Autodesk Fusion 360 part; units mm, degrees
(part 2 of 3)
  spline S18 degree 5 poles (-4.419, 9.1361) (-4.4209, 9.1399) (-4.4247, 9.1474) (-4.4306, 9.1586) (-4.439, 9.1732) (-4.4502, 9.1911) (-4.4619, 9.2087) (-4.4739, 9.2262) (-4.4861, 9.2436) (-4.4984, 9.2609) (-4.5108, 9.2782) (-4.5234, 9.2954) (-4.5362, 9.3124) (-4.5493, 9.3294) (-4.5626, 9.3462) (-4.5761, 9.3629) (-4.5898, 9.3794) (-4.6036, 9.3959) (-4.6176, 9.4123) (-4.6318, 9.4286) (-4.6461, 9.4449) (-4.6605, 9.461) (-4.6751, 9.4771) (-4.6898, 9.4931) (-4.7046, 9.509) (-4.7196, 9.5248) (-4.7348, 9.5406) (-4.75, 9.5562) (-4.7654, 9.5718) (-4.7809, 9.5873) (-4.7966, 9.6027) (-4.8123, 9.6181) (-4.8282, 9.6334) (-4.8442, 9.6486) (-4.8603, 9.6637) (-4.8765, 9.6788) (-4.8929, 9.6938) (-4.9093, 9.7087) (-4.9259, 9.7236) (-4.9425, 9.7384) (-4.9593, 9.7531) (-4.9762, 9.7677) (-4.9931, 9.7823) (-5.0102, 9.7968) (-5.0274, 9.8112) (-5.0447, 9.8256) (-5.0621, 9.8399) (-5.0796, 9.8541) (-5.0971, 9.8683) (-5.1148, 9.8824) (-5.1326, 9.8964) (-5.1505, 9.9103) (-5.1684, 9.9242) (-5.1865, 9.9381) (-5.2046, 9.9518) (-5.2229, 9.9655) (-5.2412, 9.9791) (-5.2596, 9.9927) (-5.2781, 10.0062) (-5.2967, 10.0196) (-5.3154, 10.033) (-5.3342, 10.0463) (-5.353, 10.0595) (-5.3719, 10.0727) (-5.391, 10.0858) (-5.4101, 10.0988) (-5.4293, 10.1118) (-5.4486, 10.1247) (-5.4679, 10.1375) (-5.4874, 10.1503) (-5.5069, 10.163) (-5.5226, 10.1731) (-5.5344, 10.1807) (-5.5422, 10.1857) (-5.5462, 10.1882) knots 0 0 0 0 0 0 0.01428571 0.02857143 0.04285714 0.05714286 0.07142857 0.08571429 0.1 0.11428571 0.12857143 0.14285714 0.15714286 0.17142857 0.18571429 0.2 0.21428571 0.22857143 0.24285714 0.25714286 0.27142857 0.28571429 0.3 0.31428571 0.32857143 0.34285714 0.35714286 0.37142857 0.38571429 0.4 0.41428571 0.42857143 0.44285714 0.45714286 0.47142857 0.48571429 0.5 0.51428571 0.52857143 0.54285714 0.55714286 0.57142857 0.58571429 0.6 0.61428571 0.62857143 0.64285714 0.65714286 0.67142857 0.68571429 0.7 0.71428571 0.72857143 0.74285714 0.75714286 0.77142857 0.78571429 0.8 0.81428571 0.82857143 0.84285714 0.85714286 0.87142857 0.88571429 0.9 0.91428571 0.92857143 0.94285714 0.95714286 0.97142857 0.98571429 1 1 1 1 1 1
  arc A38 (-5.5462, 10.1882) -> (-6.0502, 9.8972) centre (0, 0) ccw
  spline S19 degree 5 poles (-6.0502, 9.8972) (-6.05, 9.8926) (-6.0496, 9.8832) (-6.0489, 9.8692) (-6.048, 9.8506) (-6.0467, 9.8273) (-6.0454, 9.8041) (-6.044, 9.7809) (-6.0424, 9.7578) (-6.0408, 9.7347) (-6.039, 9.7116) (-6.0372, 9.6886) (-6.0353, 9.6656) (-6.0333, 9.6426) (-6.0311, 9.6197) (-6.0289, 9.5969) (-6.0266, 9.5741) (-6.0241, 9.5513) (-6.0216, 9.5286) (-6.019, 9.5059) (-6.0162, 9.4832) (-6.0134, 9.4606) (-6.0104, 9.4381) (-6.0074, 9.4156) (-6.0042, 9.3931) (-6.001, 9.3707) (-5.9976, 9.3484) (-5.9941, 9.3261) (-5.9905, 9.3038) (-5.9868, 9.2816) (-5.9831, 9.2595) (-5.9791, 9.2374) (-5.9751, 9.2153) (-5.971, 9.1933) (-5.9668, 9.1714) (-5.9624, 9.1495) (-5.9579, 9.1277) (-5.9533, 9.1059) (-5.9486, 9.0842) (-5.9438, 9.0626) (-5.9389, 9.041) (-5.9338, 9.0195) (-5.9287, 8.998) (-5.9234, 8.9767) (-5.9179, 8.9553) (-5.9124, 8.9341) (-5.9067, 8.9129) (-5.9009, 8.8918) (-5.895, 8.8707) (-5.8889, 8.8497) (-5.8827, 8.8288) (-5.8764, 8.808) (-5.8699, 8.7873) (-5.8632, 8.7666) (-5.8565, 8.7461) (-5.8495, 8.7256) (-5.8425, 8.7052) (-5.8353, 8.6848) (-5.8279, 8.6646) (-5.8204, 8.6444) (-5.8128, 8.6244) (-5.8048, 8.6045) (-5.7967, 8.5847) (-5.7883, 8.5651) (-5.7797, 8.5456) (-5.771, 8.5262) (-5.7622, 8.5068) (-5.7532, 8.4876) (-5.7441, 8.4685) (-5.7346, 8.4495) (-5.7247, 8.4309) (-5.7163, 8.4163) (-5.7095, 8.4056) (-5.7049, 8.3985) (-5.7025, 8.395) knots -1 -1 -1 -1 -1 -1 -0.98571429 -0.97142857 -0.95714286 -0.94285714 -0.92857143 -0.91428571 -0.9 -0.88571429 -0.87142857 -0.85714286 -0.84285714 -0.82857143 -0.81428571 -0.8 -0.78571429 -0.77142857 -0.75714286 -0.74285714 -0.72857143 -0.71428571 -0.7 -0.68571429 -0.67142857 -0.65714286 -0.64285714 -0.62857143 -0.61428571 -0.6 -0.58571429 -0.57142857 -0.55714286 -0.54285714 -0.52857143 -0.51428571 -0.5 -0.48571429 -0.47142857 -0.45714286 -0.44285714 -0.42857143 -0.41428571 -0.4 -0.38571429 -0.37142857 -0.35714286 -0.34285714 -0.32857143 -0.31428571 -0.3 -0.28571429 -0.27142857 -0.25714286 -0.24285714 -0.22857143 -0.21428571 -0.2 -0.18571429 -0.17142857 -0.15714286 -0.14285714 -0.12857143 -0.11428571 -0.1 -0.08571429 -0.07142857 -0.05714286 -0.04285714 -0.02857143 -0.01428571 0 0 0 0 0 0
  line L19 (-5.7025, 8.395) -> (-5.5568, 8.1795)
  arc A39 (-5.5826, 8.0414) -> (-5.5568, 8.1795) centre (-5.6396, 8.1235) ccw
  arc A40 (-5.5826, 8.0414) -> (-6.1024, 7.6543) centre (0, 0) ccw
  arc A41 (-6.2422, 7.6692) -> (-6.1024, 7.6543) centre (-6.1648, 7.7325) ccw
  line L20 (-6.2422, 7.6692) -> (-6.4069, 7.8707)
  spline S20 degree 5 poles (-6.4069, 7.8707) (-6.4095, 7.874) (-6.4149, 7.8804) (-6.4233, 7.8899) (-6.4348, 7.9022) (-6.4498, 7.9171) (-6.4653, 7.9315) (-6.481, 7.9458) (-6.4969, 7.9599) (-6.5128, 7.9739) (-6.5289, 7.9878) (-6.5451, 8.0016) (-6.5615, 8.0153) (-6.5781, 8.0288) (-6.5949, 8.0421) (-6.6119, 8.0552) (-6.6291, 8.0681) (-6.6464, 8.081) (-6.6638, 8.0937) (-6.6813, 8.1063) (-6.699, 8.1188) (-6.7167, 8.1312) (-6.7346, 8.1435) (-6.7526, 8.1557) (-6.7707, 8.1677) (-6.789, 8.1797) (-6.8073, 8.1915) (-6.8258, 8.2032) (-6.8444, 8.2148) (-6.8631, 8.2263) (-6.8818, 8.2377) (-6.9007, 8.249) (-6.9197, 8.2603) (-6.9387, 8.2714) (-6.9579, 8.2824) (-6.9772, 8.2933) (-6.9965, 8.3041) (-7.016, 8.3149) (-7.0355, 8.3255) (-7.0551, 8.336) (-7.0748, 8.3465) (-7.0946, 8.3568) (-7.1145, 8.3671) (-7.1345, 8.3773) (-7.1545, 8.3873) (-7.1746, 8.3973) (-7.1949, 8.4072) (-7.2152, 8.4171) (-7.2355, 8.4268) (-7.256, 8.4364) (-7.2765, 8.446) (-7.2971, 8.4554) (-7.3178, 8.4648) (-7.3385, 8.4741) (-7.3594, 8.4833) (-7.3803, 8.4924) (-7.4012, 8.5014) (-7.4223, 8.5104) (-7.4434, 8.5193) (-7.4646, 8.528) (-7.4859, 8.5367) (-7.5072, 8.5453) (-7.5286, 8.5539) (-7.5501, 8.5623) (-7.5716, 8.5707) (-7.5932, 8.5789) (-7.6149, 8.5871) (-7.6366, 8.5952) (-7.6584, 8.6033) (-7.6803, 8.6112) (-7.7022, 8.6191) (-7.7198, 8.6253) (-7.733, 8.63) (-7.7418, 8.633) (-7.7462, 8.6346) knots 0 0 0 0 0 0 0.01428571 0.02857143 0.04285714 0.05714286 0.07142857 0.08571429 0.1 0.11428571 0.12857143 0.14285714 0.15714286 0.17142857 0.18571429 0.2 0.21428571 0.22857143 0.24285714 0.25714286 0.27142857 0.28571429 0.3 0.31428571 0.32857143 0.34285714 0.35714286 0.37142857 0.38571429 0.4 0.41428571 0.42857143 0.44285714 0.45714286 0.47142857 0.48571429 0.5 0.51428571 0.52857143 0.54285714 0.55714286 0.57142857 0.58571429 0.6 0.61428571 0.62857143 0.64285714 0.65714286 0.67142857 0.68571429 0.7 0.71428571 0.72857143 0.74285714 0.75714286 0.77142857 0.78571429 0.8 0.81428571 0.82857143 0.84285714 0.85714286 0.87142857 0.88571429 0.9 0.91428571 0.92857143 0.94285714 0.95714286 0.97142857 0.98571429 1 1 1 1 1 1
  arc A42 (-7.7462, 8.6346) -> (-8.1696, 8.2352) centre (0, 0) ccw
  spline S21 degree 5 poles (-8.1696, 8.2352) (-8.1683, 8.2307) (-8.1657, 8.2217) (-8.1619, 8.2082) (-8.1567, 8.1903) (-8.1501, 8.168) (-8.1434, 8.1457) (-8.1367, 8.1234) (-8.1298, 8.1013) (-8.1229, 8.0792) (-8.1159, 8.0571) (-8.1088, 8.0351) (-8.1016, 8.0132) (-8.0944, 7.9914) (-8.087, 7.9696) (-8.0796, 7.9478) (-8.072, 7.9262) (-8.0644, 7.9046) (-8.0567, 7.883) (-8.0489, 7.8616) (-8.041, 7.8402) (-8.0331, 7.8189) (-8.025, 7.7976) (-8.0168, 7.7764) (-8.0086, 7.7553) (-8.0002, 7.7342) (-7.9918, 7.7133) (-7.9833, 7.6924) (-7.9747, 7.6715) (-7.966, 7.6508) (-7.9572, 7.6301) (-7.9483, 7.6095) (-7.9393, 7.589) (-7.9302, 7.5685) (-7.921, 7.5482) (-7.9117, 7.5279) (-7.9023, 7.5077) (-7.8928, 7.4876) (-7.8833, 7.4675) (-7.8736, 7.4476) (-7.8638, 7.4277) (-7.8539, 7.4079) (-7.8439, 7.3883) (-7.8339, 7.3687) (-7.8237, 7.3492) (-7.8133, 7.3298) (-7.8029, 7.3105) (-7.7924, 7.2912) (-7.7818, 7.2721) (-7.7711, 7.2531) (-7.7602, 7.2342) (-7.7492, 7.2154) (-7.7381, 7.1967) (-7.7269, 7.1782) (-7.7156, 7.1597) (-7.7041, 7.1414) (-7.6925, 7.1231) (-7.6808, 7.105) (-7.669, 7.087) (-7.6571, 7.0691) (-7.645, 7.0514) (-7.6327, 7.0338) (-7.6202, 7.0165) (-7.6075, 6.9993) (-7.5947, 6.9823) (-7.5817, 6.9655) (-7.5687, 6.9487) (-7.5555, 6.932) (-7.5422, 6.9155) (-7.5287, 6.8993) (-7.5147, 6.8834) (-7.5031, 6.8712) (-7.4941, 6.8623) (-7.488, 6.8565) (-7.4849, 6.8537) knots -1 -1 -1 -1 -1 -1 -0.98571429 -0.97142857 -0.95714286 -0.94285714 -0.92857143 -0.91428571 -0.9 -0.88571429 -0.87142857 -0.85714286 -0.84285714 -0.82857143 -0.81428571 -0.8 -0.78571429 -0.77142857 -0.75714286 -0.74285714 -0.72857143 -0.71428571 -0.7 -0.68571429 -0.67142857 -0.65714286 -0.64285714 -0.62857143 -0.61428571 -0.6 -0.58571429 -0.57142857 -0.55714286 -0.54285714 -0.52857143 -0.51428571 -0.5 -0.48571429 -0.47142857 -0.45714286 -0.44285714 -0.42857143 -0.41428571 -0.4 -0.38571429 -0.37142857 -0.35714286 -0.34285714 -0.32857143 -0.31428571 -0.3 -0.28571429 -0.27142857 -0.25714286 -0.24285714 -0.22857143 -0.21428571 -0.2 -0.18571429 -0.17142857 -0.15714286 -0.14285714 -0.12857143 -0.11428571 -0.1 -0.08571429 -0.07142857 -0.05714286 -0.04285714 -0.02857143 -0.01428571 0 0 0 0 0 0
  line L21 (-7.4849, 6.8537) -> (-7.2933, 6.6776)
  arc A43 (-7.2866, 6.5372) -> (-7.2933, 6.6776) centre (-7.361, 6.6039) ccw
  arc A44 (-7.2866, 6.5372) -> (-7.7031, 6.0407) centre (0, 0) ccw
  arc A45 (-7.8426, 6.023) -> (-7.7031, 6.0407) centre (-7.7818, 6.1024) ccw
  line L22 (-7.8426, 6.023) -> (-8.0493, 6.181)
  spline S22 degree 5 poles (-8.0493, 6.181) (-8.0526, 6.1836) (-8.0594, 6.1886) (-8.0697, 6.196) (-8.0837, 6.2052) (-8.1018, 6.2162) (-8.1201, 6.2268) (-8.1387, 6.237) (-8.1574, 6.247) (-8.1762, 6.257) (-8.1951, 6.2668) (-8.214, 6.2765) (-8.2331, 6.286) (-8.2524, 6.2953) (-8.2718, 6.3044) (-8.2914, 6.3132) (-8.311, 6.3219) (-8.3308, 6.3304) (-8.3507, 6.3387) (-8.3707, 6.347) (-8.3907, 6.3551) (-8.4109, 6.3631) (-8.4311, 6.3709) (-8.4514, 6.3786) (-8.4718, 6.3861) (-8.4923, 6.3935) (-8.5129, 6.4008) (-8.5336, 6.4079) (-8.5544, 6.4149) (-8.5752, 6.4218) (-8.5961, 6.4286) (-8.6171, 6.4353) (-8.6381, 6.4418) (-8.6592, 6.4482) (-8.6804, 6.4545) (-8.7017, 6.4607) (-8.723, 6.4668) (-8.7444, 6.4727) (-8.7658, 6.4786) (-8.7874, 6.4843) (-8.809, 6.4899) (-8.8306, 6.4954) (-8.8523, 6.5008) (-8.8741, 6.5061) (-8.8959, 6.5113) (-8.9178, 6.5164) (-8.9398, 6.5214) (-8.9618, 6.5262) (-8.9838, 6.531) (-9.006, 6.5357) (-9.0281, 6.5402) (-9.0504, 6.5447) (-9.0727, 6.549) (-9.095, 6.5533) (-9.1174, 6.5574) (-9.1398, 6.5615) (-9.1623, 6.5654) (-9.1849, 6.5693) (-9.2075, 6.573) (-9.2301, 6.5767) (-9.2528, 6.5803) (-9.2755, 6.5837) (-9.2983, 6.5871) (-9.3212, 6.5903) (-9.344, 6.5935) (-9.367, 6.5966) (-9.3899, 6.5996) (-9.413, 6.6024) (-9.436, 6.6052) (-9.4591, 6.6079) (-9.4823, 6.6105) (-9.5008, 6.6125) (-9.5148, 6.614) (-9.5241, 6.6149) (-9.5287, 6.6154) knots 0 0 0 0 0 0 0.01428571 0.02857143 0.04285714 0.05714286 0.07142857 0.08571429 0.1 0.11428571 0.12857143 0.14285714 0.15714286 0.17142857 0.18571429 0.2 0.21428571 0.22857143 0.24285714 0.25714286 0.27142857 0.28571429 0.3 0.31428571 0.32857143 0.34285714 0.35714286 0.37142857 0.38571429 0.4 0.41428571 0.42857143 0.44285714 0.45714286 0.47142857 0.48571429 0.5 0.51428571 0.52857143 0.54285714 0.55714286 0.57142857 0.58571429 0.6 0.61428571 0.62857143 0.64285714 0.65714286 0.67142857 0.68571429 0.7 0.71428571 0.72857143 0.74285714 0.75714286 0.77142857 0.78571429 0.8 0.81428571 0.82857143 0.84285714 0.85714286 0.87142857 0.88571429 0.9 0.91428571 0.92857143 0.94285714 0.95714286 0.97142857 0.98571429 1 1 1 1 1 1
  arc A46 (-9.5287, 6.6154) -> (-9.8485, 6.1292) centre (0, 0) ccw
  spline S23 degree 5 poles (-9.8485, 6.1292) (-9.8462, 6.1251) (-9.8417, 6.1169) (-9.8348, 6.1047) (-9.8256, 6.0885) (-9.8141, 6.0683) (-9.8024, 6.0481) (-9.7907, 6.028) (-9.779, 6.008) (-9.7672, 5.9881) (-9.7553, 5.9683) (-9.7433, 5.9485) (-9.7312, 5.9289) (-9.7191, 5.9093) (-9.7069, 5.8898) (-9.6947, 5.8703) (-9.6824, 5.851) (-9.67, 5.8317) (-9.6575, 5.8125) (-9.645, 5.7935) (-9.6324, 5.7745) (-9.6197, 5.7555) (-9.6069, 5.7367) (-9.5941, 5.718) (-9.5812, 5.6993) (-9.5682, 5.6808) (-9.5552, 5.6623) (-9.5421, 5.6439) (-9.5289, 5.6257) (-9.5156, 5.6075) (-9.5023, 5.5894) (-9.4889, 5.5714) (-9.4754, 5.5535) (-9.4618, 5.5357) (-9.4482, 5.518) (-9.4345, 5.5004) (-9.4207, 5.4829) (-9.4068, 5.4655) (-9.3929, 5.4482) (-9.3789, 5.431) (-9.3648, 5.414) (-9.3506, 5.397) (-9.3364, 5.3802) (-9.322, 5.3634) (-9.3076, 5.3468) (-9.2931, 5.3303) (-9.2785, 5.3139) (-9.2639, 5.2976) (-9.2491, 5.2815) (-9.2343, 5.2655) (-9.2194, 5.2496) (-9.2044, 5.2338) (-9.1892, 5.2182) (-9.174, 5.2027) (-9.1587, 5.1874) (-9.1434, 5.1722) (-9.1279, 5.1571) (-9.1123, 5.1422) (-9.0967, 5.1274) (-9.0809, 5.1127) (-9.0651, 5.0983) (-9.0491, 5.084) (-9.0329, 5.07) (-9.0166, 5.0562) (-9.0002, 5.0427) (-8.9837, 5.0292) (-8.9671, 5.0159) (-8.9505, 5.0028) (-8.9337, 4.9897) (-8.9168, 4.9771) (-8.8996, 4.9649) (-8.8855, 4.9556) (-8.8747, 4.9491) (-8.8673, 4.9448) (-8.8637, 4.9428) knots -1 -1 -1 -1 -1 -1 -0.98571429 -0.97142857 -0.95714286 -0.94285714 -0.92857143 -0.91428571 -0.9 -0.88571429 -0.87142857 -0.85714286 -0.84285714 -0.82857143 -0.81428571 -0.8 -0.78571429 -0.77142857 -0.75714286 -0.74285714 -0.72857143 -0.71428571 -0.7 -0.68571429 -0.67142857 -0.65714286 -0.64285714 -0.62857143 -0.61428571 -0.6 -0.58571429 -0.57142857 -0.55714286 -0.54285714 -0.52857143 -0.51428571 -0.5 -0.48571429 -0.47142857 -0.45714286 -0.44285714 -0.42857143 -0.41428571 -0.4 -0.38571429 -0.37142857 -0.35714286 -0.34285714 -0.32857143 -0.31428571 -0.3 -0.28571429 -0.27142857 -0.25714286 -0.24285714 -0.22857143 -0.21428571 -0.2 -0.18571429 -0.17142857 -0.15714286 -0.14285714 -0.12857143 -0.11428571 -0.1 -0.08571429 -0.07142857 -0.05714286 -0.04285714 -0.02857143 -0.01428571 0 0 0 0 0 0
  line L23 (-8.8637, 4.9428) -> (-8.6367, 4.8156)
  arc A47 (-8.5977, 4.6806) -> (-8.6367, 4.8156) centre (-8.6855, 4.7284) ccw
  arc A48 (-8.5977, 4.6806) -> (-8.8886, 4.1014) centre (0, 0) ccw
  arc A49 (-9.0202, 4.052) -> (-8.8886, 4.1014) centre (-8.9794, 4.1433) ccw
  line L24 (-9.0202, 4.052) -> (-9.2577, 4.1581)
  spline S24 degree 5 poles (-9.2577, 4.1581) (-9.2616, 4.1598) (-9.2693, 4.1632) (-9.281, 4.1679) (-9.2969, 4.1737) (-9.317, 4.1803) (-9.3372, 4.1863) (-9.3577, 4.1919) (-9.3782, 4.1974) (-9.3988, 4.2028) (-9.4194, 4.208) (-9.4401, 4.2131) (-9.4609, 4.2179) (-9.4817, 4.2225) (-9.5027, 4.2268) (-9.5238, 4.2309) (-9.5449, 4.2348) (-9.5662, 4.2385) (-9.5874, 4.2421) (-9.6088, 4.2455) (-9.6301, 4.2487) (-9.6516, 4.2519) (-9.6731, 4.2548) (-9.6946, 4.2576) (-9.7162, 4.2602) (-9.7379, 4.2627) (-9.7596, 4.265) (-9.7814, 4.2672) (-9.8032, 4.2693) (-9.825, 4.2712) (-9.8469, 4.2729) (-9.8689, 4.2746) (-9.8908, 4.2761) (-9.9129, 4.2775) (-9.9349, 4.2787) (-9.9571, 4.2798) (-9.9792, 4.2808) (-10.0014, 4.2817) (-10.0236, 4.2824) (-10.0459, 4.283) (-10.0682, 4.2835) (-10.0905, 4.2839) (-10.1129, 4.2841) (-10.1353, 4.2843) (-10.1577, 4.2843) (-10.1802, 4.2842) (-10.2027, 4.2839) (-10.2253, 4.2836) (-10.2478, 4.2831) (-10.2704, 4.2826) (-10.2931, 4.2819) (-10.3157, 4.2811) (-10.3384, 4.2802) (-10.3611, 4.2792) (-10.3839, 4.2781) (-10.4066, 4.2768) (-10.4294, 4.2755) (-10.4523, 4.274) (-10.4751, 4.2725) (-10.498, 4.2708) (-10.5209, 4.269) (-10.5438, 4.2672) (-10.5668, 4.2652) (-10.5897, 4.2631) (-10.6127, 4.2609) (-10.6358, 4.2586) (-10.6588, 4.2562) (-10.6819, 4.2537) (-10.7049, 4.2511) (-10.728, 4.2484) (-10.7512, 4.2456) (-10.7697, 4.2432) (-10.7836, 4.2414) (-10.7928, 4.2402) (-10.7975, 4.2396) knots 0 0 0 0 0 0 0.01428571 0.02857143 0.04285714 0.05714286 0.07142857 0.08571429 0.1 0.11428571 0.12857143 0.14285714 0.15714286 0.17142857 0.18571429 0.2 0.21428571 0.22857143 0.24285714 0.25714286 0.27142857 0.28571429 0.3 0.31428571 0.32857143 0.34285714 0.35714286 0.37142857 0.38571429 0.4 0.41428571 0.42857143 0.44285714 0.45714286 0.47142857 0.48571429 0.5 0.51428571 0.52857143 0.54285714 0.55714286 0.57142857 0.58571429 0.6 0.61428571 0.62857143 0.64285714 0.65714286 0.67142857 0.68571429 0.7 0.71428571 0.72857143 0.74285714 0.75714286 0.77142857 0.78571429 0.8 0.81428571 0.82857143 0.84285714 0.85714286 0.87142857 0.88571429 0.9 0.91428571 0.92857143 0.94285714 0.95714286 0.97142857 0.98571429 1 1 1 1 1 1
  arc A50 (-10.7975, 4.2396) -> (-10.9965, 3.6928) centre (0, 0) ccw
  spline S25 degree 5 poles (-10.9965, 3.6928) (-10.9934, 3.6893) (-10.9871, 3.6824) (-10.9776, 3.6721) (-10.9649, 3.6584) (-10.949, 3.6414) (-10.933, 3.6245) (-10.917, 3.6076) (-10.9009, 3.5909) (-10.8848, 3.5743) (-10.8687, 3.5577) (-10.8525, 3.5412) (-10.8362, 3.5249) (-10.8199, 3.5086) (-10.8036, 3.4924) (-10.7872, 3.4763) (-10.7707, 3.4604) (-10.7542, 3.4445) (-10.7376, 3.4287) (-10.721, 3.413) (-10.7044, 3.3974) (-10.6877, 3.382) (-10.6709, 3.3666) (-10.6541, 3.3513) (-10.6373, 3.3361) (-10.6204, 3.3211) (-10.6034, 3.3061) (-10.5864, 3.2912) (-10.5694, 3.2765) (-10.5523, 3.2619) (-10.5352, 3.2473) (-10.518, 3.2329) (-10.5007, 3.2186) (-10.4834, 3.2044) (-10.4661, 3.1904) (-10.4487, 3.1764) (-10.4312, 3.1625) (-10.4137, 3.1488) (-10.3962, 3.1352) (-10.3786, 3.1217) (-10.3609, 3.1084) (-10.3432, 3.0951) (-10.3254, 3.082) (-10.3076, 3.0691) (-10.2898, 3.0562) (-10.2719, 3.0435) (-10.2539, 3.0309) (-10.2359, 3.0185) (-10.2178, 3.0061) (-10.1997, 2.994) (-10.1815, 2.9819) (-10.1632, 2.9701) (-10.1449, 2.9583) (-10.1266, 2.9468) (-10.1082, 2.9354) (-10.0897, 2.9242) (-10.0712, 2.9131) (-10.0526, 2.9021) (-10.0339, 2.8913) (-10.0152, 2.8807) (-9.9965, 2.8703) (-9.9776, 2.8601) (-9.9587, 2.8502) (-9.9396, 2.8406) (-9.9205, 2.8311) (-9.9014, 2.8219) (-9.8822, 2.8128) (-9.8629, 2.8038) (-9.8436, 2.795) (-9.8242, 2.7865) (-9.8047, 2.7786) (-9.7888, 2.7729) (-9.7768, 2.769) (-9.7687, 2.7666) (-9.7646, 2.7655) knots -1 -1 -1 -1 -1 -1 -0.98571429 -0.97142857 -0.95714286 -0.94285714 -0.92857143 -0.91428571 -0.9 -0.88571429 -0.87142857 -0.85714286 -0.84285714 -0.82857143 -0.81428571 -0.8 -0.78571429 -0.77142857 -0.75714286 -0.74285714 -0.72857143 -0.71428571 -0.7 -0.68571429 -0.67142857 -0.65714286 -0.64285714 -0.62857143 -0.61428571 -0.6 -0.58571429 -0.57142857 -0.55714286 -0.54285714 -0.52857143 -0.51428571 -0.5 -0.48571429 -0.47142857 -0.45714286 -0.44285714 -0.42857143 -0.41428571 -0.4 -0.38571429 -0.37142857 -0.35714286 -0.34285714 -0.32857143 -0.31428571 -0.3 -0.28571429 -0.27142857 -0.25714286 -0.24285714 -0.22857143 -0.21428571 -0.2 -0.18571429 -0.17142857 -0.15714286 -0.14285714 -0.12857143 -0.11428571 -0.1 -0.08571429 -0.07142857 -0.05714286 -0.04285714 -0.02857143 -0.01428571 0 0 0 0 0 0
  line L25 (-9.7646, 2.7655) -> (-9.5144, 2.6941)
  arc A51 (-9.4454, 2.5716) -> (-9.5144, 2.6941) centre (-9.5419, 2.5979) ccw
  arc A52 (-9.4454, 2.5716) -> (-9.5948, 1.941) centre (0, 0) ccw
  arc A53 (-9.7115, 1.8626) -> (-9.5948, 1.941) centre (-9.6929, 1.9608) ccw
  line L26 (-9.7115, 1.8626) -> (-9.9671, 1.9111)
  spline S26 degree 5 poles (-9.9671, 1.9111) (-9.9713, 1.9118) (-9.9796, 1.9133) (-9.9921, 1.9152) (-10.0088, 1.9172) (-10.0299, 1.919) (-10.051, 1.9201) (-10.0722, 1.9209) (-10.0934, 1.9215) (-10.1146, 1.922) (-10.1359, 1.9223) (-10.1572, 1.9225) (-10.1786, 1.9224) (-10.1999, 1.922) (-10.2214, 1.9214) (-10.2428, 1.9206) (-10.2643, 1.9195) (-10.2858, 1.9182) (-10.3073, 1.9167) (-10.3288, 1.9151) (-10.3504, 1.9134) (-10.372, 1.9114) (-10.3936, 1.9094) (-10.4152, 1.9071) (-10.4368, 1.9047) (-10.4584, 1.9021) (-10.4801, 1.8994) (-10.5018, 1.8965) (-10.5235, 1.8934) (-10.5452, 1.8902) (-10.5669, 1.8869) (-10.5886, 1.8835) (-10.6104, 1.8798) (-10.6321, 1.8761) (-10.6539, 1.8722) (-10.6757, 1.8682) (-10.6974, 1.8641) (-10.7192, 1.8598) (-10.741, 1.8554) (-10.7628, 1.8508) (-10.7846, 1.8462) (-10.8065, 1.8414) (-10.8283, 1.8364) (-10.8501, 1.8314) (-10.872, 1.8262) (-10.8938, 1.821) (-10.9157, 1.8156) (-10.9375, 1.81) (-10.9594, 1.8044) (-10.9812, 1.7986) (-11.0031, 1.7927) (-11.0249, 1.7867) (-11.0468, 1.7806) (-11.0687, 1.7744) (-11.0906, 1.7681) (-11.1124, 1.7616) (-11.1343, 1.7551) (-11.1562, 1.7484) (-11.1781, 1.7416) (-11.1999, 1.7347) (-11.2218, 1.7277) (-11.2437, 1.7206) (-11.2656, 1.7133) (-11.2874, 1.706) (-11.3093, 1.6986) (-11.3312, 1.691) (-11.353, 1.6834) (-11.3749, 1.6756) (-11.3968, 1.6678) (-11.4186, 1.6598) (-11.4405, 1.6517) (-11.4579, 1.6452) (-11.4711, 1.6403) (-11.4798, 1.6369) (-11.4842, 1.6353) knots 0 0 0 0 0 0 0.01428571 0.02857143 0.04285714 0.05714286 0.07142857 0.08571429 0.1 0.11428571 0.12857143 0.14285714 0.15714286 0.17142857 0.18571429 0.2 0.21428571 0.22857143 0.24285714 0.25714286 0.27142857 0.28571429 0.3 0.31428571 0.32857143 0.34285714 0.35714286 0.37142857 0.38571429 0.4 0.41428571 0.42857143 0.44285714 0.45714286 0.47142857 0.48571429 0.5 0.51428571 0.52857143 0.54285714 0.55714286 0.57142857 0.58571429 0.6 0.61428571 0.62857143 0.64285714 0.65714286 0.67142857 0.68571429 0.7 0.71428571 0.72857143 0.74285714 0.75714286 0.77142857 0.78571429 0.8 0.81428571 0.82857143 0.84285714 0.85714286 0.87142857 0.88571429 0.9 0.91428571 0.92857143 0.94285714 0.95714286 0.97142857 0.98571429 1 1 1 1 1 1
  arc A54 (-11.4842, 1.6353) -> (-11.5517, 1.0572) centre (0, 0) ccw
  spline S27 degree 5 poles (-11.5517, 1.0572) (-11.5479, 1.0546) (-11.5401, 1.0494) (-11.5285, 1.0415) (-11.513, 1.0311) (-11.4936, 1.0182) (-11.4742, 1.0055) (-11.4547, 0.9928) (-11.4352, 0.9802) (-11.4157, 0.9677) (-11.3962, 0.9553) (-11.3766, 0.943) (-11.357, 0.9309) (-11.3374, 0.9188) (-11.3178, 0.9068) (-11.2981, 0.8949) (-11.2784, 0.8832) (-11.2587, 0.8715) (-11.2389, 0.86) (-11.2192, 0.8486) (-11.1994, 0.8373) (-11.1795, 0.826) (-11.1597, 0.8149) (-11.1398, 0.8039) (-11.1199, 0.7931) (-11.1, 0.7823) (-11.0801, 0.7717) (-11.0601, 0.7611) (-11.0401, 0.7507) (-11.0201, 0.7404) (-11.0001, 0.7302) (-10.98, 0.7202) (-10.9599, 0.7102) (-10.9398, 0.7004) (-10.9197, 0.6907) (-10.8995, 0.6811) (-10.8794, 0.6717) (-10.8592, 0.6624) (-10.839, 0.6532) (-10.8187, 0.6441) (-10.7985, 0.6352) (-10.7782, 0.6264) (-10.7579, 0.6177) (-10.7376, 0.6092) (-10.7172, 0.6008) (-10.6969, 0.5926) (-10.6765, 0.5845) (-10.6561, 0.5765) (-10.6356, 0.5687) (-10.6152, 0.5611) (-10.5947, 0.5535) (-10.5742, 0.5462) (-10.5537, 0.539) (-10.5332, 0.532) (-10.5126, 0.5252) (-10.4921, 0.5185) (-10.4715, 0.512) (-10.4509, 0.5056) (-10.4303, 0.4994) (-10.4096, 0.4934) (-10.389, 0.4876) (-10.3683, 0.482) (-10.3475, 0.4768) (-10.3268, 0.4718) (-10.306, 0.467) (-10.2852, 0.4624) (-10.2645, 0.458) (-10.2437, 0.4537) (-10.2229, 0.4496) (-10.202, 0.4458) (-10.1812, 0.4426) (-10.1644, 0.4407) (-10.1518, 0.4397) (-10.1434, 0.4392) (-10.1392, 0.439) knots -1 -1 -1 -1 -1 -1 -0.98571429 -0.97142857 -0.95714286 -0.94285714 -0.92857143 -0.91428571 -0.9 -0.88571429 -0.87142857 -0.85714286 -0.84285714 -0.82857143 -0.81428571 -0.8 -0.78571429 -0.77142857 -0.75714286 -0.74285714 -0.72857143 -0.71428571 -0.7 -0.68571429 -0.67142857 -0.65714286 -0.64285714 -0.62857143 -0.61428571 -0.6 -0.58571429 -0.57142857 -0.55714286 -0.54285714 -0.52857143 -0.51428571 -0.5 -0.48571429 -0.47142857 -0.45714286 -0.44285714 -0.42857143 -0.41428571 -0.4 -0.38571429 -0.37142857 -0.35714286 -0.34285714 -0.32857143 -0.31428571 -0.3 -0.28571429 -0.27142857 -0.25714286 -0.24285714 -0.22857143 -0.21428571 -0.2 -0.18571429 -0.17142857 -0.15714286 -0.14285714 -0.12857143 -0.11428571 -0.1 -0.08571429 -0.07142857 -0.05714286 -0.04285714 -0.02857143 -0.01428571 0 0 0 0 0 0
  line L27 (-10.1392, 0.439) -> (-9.8793, 0.4273)
  arc A55 (-9.7838, 0.3241) -> (-9.8793, 0.4273) centre (-9.8838, 0.3274) ccw
  arc A56 (-9.7838, 0.3241) -> (-9.7838, -0.3241) centre (0, 0) ccw
  arc A57 (-9.8793, -0.4273) -> (-9.7838, -0.3241) centre (-9.8838, -0.3274) ccw
  line L28 (-9.8793, -0.4273) -> (-10.1392, -0.439)
  spline S28 degree 5 poles (-10.1392, -0.439) (-10.1434, -0.4392) (-10.1518, -0.4397) (-10.1644, -0.4407) (-10.1812, -0.4426) (-10.202, -0.4458) (-10.2229, -0.4496) (-10.2437, -0.4537) (-10.2645, -0.458) (-10.2852, -0.4624) (-10.306, -0.467) (-10.3268, -0.4718) (-10.3475, -0.4768) (-10.3683, -0.482) (-10.389, -0.4876) (-10.4096, -0.4934) (-10.4303, -0.4994) (-10.4509, -0.5056) (-10.4715, -0.512) (-10.4921, -0.5185) (-10.5126, -0.5252) (-10.5332, -0.532) (-10.5537, -0.539) (-10.5742, -0.5462) (-10.5947, -0.5535) (-10.6152, -0.5611) (-10.6356, -0.5687) (-10.6561, -0.5765) (-10.6765, -0.5845) (-10.6969, -0.5926) (-10.7172, -0.6008) (-10.7376, -0.6092) (-10.7579, -0.6177) (-10.7782, -0.6264) (-10.7985, -0.6352) (-10.8187, -0.6441) (-10.839, -0.6532) (-10.8592, -0.6624) (-10.8794, -0.6717) (-10.8995, -0.6811) (-10.9197, -0.6907) (-10.9398, -0.7004) (-10.9599, -0.7102) (-10.98, -0.7202) (-11.0001, -0.7302) (-11.0201, -0.7404) (-11.0401, -0.7507) (-11.0601, -0.7611) (-11.0801, -0.7717) (-11.1, -0.7823) (-11.1199, -0.7931) (-11.1398, -0.8039) (-11.1597, -0.8149) (-11.1795, -0.826) (-11.1994, -0.8373) (-11.2192, -0.8486) (-11.2389, -0.86) (-11.2587, -0.8715) (-11.2784, -0.8832) (-11.2981, -0.8949) (-11.3178, -0.9068) (-11.3374, -0.9188) (-11.357, -0.9309) (-11.3766, -0.943) (-11.3962, -0.9553) (-11.4157, -0.9677) (-11.4352, -0.9802) (-11.4547, -0.9928) (-11.4742, -1.0055) (-11.4936, -1.0182) (-11.513, -1.0311) (-11.5285, -1.0415) (-11.5401, -1.0494) (-11.5479, -1.0546) (-11.5517, -1.0572) knots 0 0 0 0 0 0 0.01428571 0.02857143 0.04285714 0.05714286 0.07142857 0.08571429 0.1 0.11428571 0.12857143 0.14285714 0.15714286 0.17142857 0.18571429 0.2 0.21428571 0.22857143 0.24285714 0.25714286 0.27142857 0.28571429 0.3 0.31428571 0.32857143 0.34285714 0.35714286 0.37142857 0.38571429 0.4 0.41428571 0.42857143 0.44285714 0.45714286 0.47142857 0.48571429 0.5 0.51428571 0.52857143 0.54285714 0.55714286 0.57142857 0.58571429 0.6 0.61428571 0.62857143 0.64285714 0.65714286 0.67142857 0.68571429 0.7 0.71428571 0.72857143 0.74285714 0.75714286 0.77142857 0.78571429 0.8 0.81428571 0.82857143 0.84285714 0.85714286 0.87142857 0.88571429 0.9 0.91428571 0.92857143 0.94285714 0.95714286 0.97142857 0.98571429 1 1 1 1 1 1
  arc A58 (-11.5517, -1.0572) -> (-11.4842, -1.6353) centre (0, 0) ccw
  spline S29 degree 5 poles (-11.4842, -1.6353) (-11.4798, -1.6369) (-11.4711, -1.6403) (-11.4579, -1.6452) (-11.4405, -1.6517) (-11.4186, -1.6598) (-11.3968, -1.6678) (-11.3749, -1.6756) (-11.353, -1.6834) (-11.3312, -1.691) (-11.3093, -1.6986) (-11.2874, -1.706) (-11.2656, -1.7133) (-11.2437, -1.7206) (-11.2218, -1.7277) (-11.1999, -1.7347) (-11.1781, -1.7416) (-11.1562, -1.7484) (-11.1343, -1.7551) (-11.1124, -1.7616) (-11.0906, -1.7681) (-11.0687, -1.7744) (-11.0468, -1.7806) (-11.0249, -1.7867) (-11.0031, -1.7927) (-10.9812, -1.7986) (-10.9594, -1.8044) (-10.9375, -1.81) (-10.9157, -1.8156) (-10.8938, -1.821) (-10.872, -1.8262) (-10.8501, -1.8314) (-10.8283, -1.8364) (-10.8065, -1.8414) (-10.7846, -1.8462) (-10.7628, -1.8508) (-10.741, -1.8554) (-10.7192, -1.8598) (-10.6974, -1.8641) (-10.6757, -1.8682) (-10.6539, -1.8722) (-10.6321, -1.8761) (-10.6104, -1.8798) (-10.5886, -1.8835) (-10.5669, -1.8869) (-10.5452, -1.8902) (-10.5235, -1.8934) (-10.5018, -1.8965) (-10.4801, -1.8994) (-10.4584, -1.9021) (-10.4368, -1.9047) (-10.4152, -1.9071) (-10.3936, -1.9094) (-10.372, -1.9114) (-10.3504, -1.9134) (-10.3288, -1.9151) (-10.3073, -1.9167) (-10.2858, -1.9182) (-10.2643, -1.9195) (-10.2428, -1.9206) (-10.2214, -1.9214) (-10.1999, -1.922) (-10.1786, -1.9224) (-10.1572, -1.9225) (-10.1359, -1.9223) (-10.1146, -1.922) (-10.0934, -1.9215) (-10.0722, -1.9209) (-10.051, -1.9201) (-10.0299, -1.919) (-10.0088, -1.9172) (-9.9921, -1.9152) (-9.9796, -1.9133) (-9.9713, -1.9118) (-9.9671, -1.9111) knots -1 -1 -1 -1 -1 -1 -0.98571429 -0.97142857 -0.95714286 -0.94285714 -0.92857143 -0.91428571 -0.9 -0.88571429 -0.87142857 -0.85714286 -0.84285714 -0.82857143 -0.81428571 -0.8 -0.78571429 -0.77142857 -0.75714286 -0.74285714 -0.72857143 -0.71428571 -0.7 -0.68571429 -0.67142857 -0.65714286 -0.64285714 -0.62857143 -0.61428571 -0.6 -0.58571429 -0.57142857 -0.55714286 -0.54285714 -0.52857143 -0.51428571 -0.5 -0.48571429 -0.47142857 -0.45714286 -0.44285714 -0.42857143 -0.41428571 -0.4 -0.38571429 -0.37142857 -0.35714286 -0.34285714 -0.32857143 -0.31428571 -0.3 -0.28571429 -0.27142857 -0.25714286 -0.24285714 -0.22857143 -0.21428571 -0.2 -0.18571429 -0.17142857 -0.15714286 -0.14285714 -0.12857143 -0.11428571 -0.1 -0.08571429 -0.07142857 -0.05714286 -0.04285714 -0.02857143 -0.01428571 0 0 0 0 0 0
  line L29 (-9.9671, -1.9111) -> (-9.7115, -1.8626)
  arc A59 (-9.5948, -1.941) -> (-9.7115, -1.8626) centre (-9.6929, -1.9608) ccw
  arc A60 (-9.5948, -1.941) -> (-9.4454, -2.5716) centre (0, 0) ccw
  arc A61 (-9.5144, -2.6941) -> (-9.4454, -2.5716) centre (-9.5419, -2.5979) ccw
  line L30 (-9.5144, -2.6941) -> (-9.7646, -2.7655)
  spline S30 degree 5 poles (-9.7646, -2.7655) (-9.7687, -2.7666) (-9.7768, -2.769) (-9.7888, -2.7729) (-9.8047, -2.7786) (-9.8242, -2.7865) (-9.8436, -2.795) (-9.8629, -2.8038) (-9.8822, -2.8128) (-9.9014, -2.8219) (-9.9205, -2.8311) (-9.9396, -2.8406) (-9.9587, -2.8502) (-9.9776, -2.8601) (-9.9965, -2.8703) (-10.0152, -2.8807) (-10.0339, -2.8913) (-10.0526, -2.9021) (-10.0712, -2.9131) (-10.0897, -2.9242) (-10.1082, -2.9354) (-10.1266, -2.9468) (-10.1449, -2.9583) (-10.1632, -2.9701) (-10.1815, -2.9819) (-10.1997, -2.994) (-10.2178, -3.0061) (-10.2359, -3.0185) (-10.2539, -3.0309) (-10.2719, -3.0435) (-10.2898, -3.0562) (-10.3076, -3.0691) (-10.3254, -3.082) (-10.3432, -3.0951) (-10.3609, -3.1084) (-10.3786, -3.1217) (-10.3962, -3.1352) (-10.4137, -3.1488) (-10.4312, -3.1625) (-10.4487, -3.1764) (-10.4661, -3.1904) (-10.4834, -3.2044) (-10.5007, -3.2186) (-10.518, -3.2329) (-10.5352, -3.2473) (-10.5523, -3.2619) (-10.5694, -3.2765) (-10.5864, -3.2912) (-10.6034, -3.3061) (-10.6204, -3.3211) (-10.6373, -3.3361) (-10.6541, -3.3513) (-10.6709, -3.3666) (-10.6877, -3.382) (-10.7044, -3.3974) (-10.721, -3.413) (-10.7376, -3.4287) (-10.7542, -3.4445) (-10.7707, -3.4604) (-10.7872, -3.4763) (-10.8036, -3.4924) (-10.8199, -3.5086) (-10.8362, -3.5249) (-10.8525, -3.5412) (-10.8687, -3.5577) (-10.8848, -3.5743) (-10.9009, -3.5909) (-10.917, -3.6076) (-10.933, -3.6245) (-10.949, -3.6414) (-10.9649, -3.6584) (-10.9776, -3.6721) (-10.9871, -3.6824) (-10.9934, -3.6893) (-10.9965, -3.6928) knots 0 0 0 0 0 0 0.01428571 0.02857143 0.04285714 0.05714286 0.07142857 0.08571429 0.1 0.11428571 0.12857143 0.14285714 0.15714286 0.17142857 0.18571429 0.2 0.21428571 0.22857143 0.24285714 0.25714286 0.27142857 0.28571429 0.3 0.31428571 0.32857143 0.34285714 0.35714286 0.37142857 0.38571429 0.4 0.41428571 0.42857143 0.44285714 0.45714286 0.47142857 0.48571429 0.5 0.51428571 0.52857143 0.54285714 0.55714286 0.57142857 0.58571429 0.6 0.61428571 0.62857143 0.64285714 0.65714286 0.67142857 0.68571429 0.7 0.71428571 0.72857143 0.74285714 0.75714286 0.77142857 0.78571429 0.8 0.81428571 0.82857143 0.84285714 0.85714286 0.87142857 0.88571429 0.9 0.91428571 0.92857143 0.94285714 0.95714286 0.97142857 0.98571429 1 1 1 1 1 1
  arc A62 (-10.9965, -3.6928) -> (-10.7975, -4.2396) centre (0, 0) ccw
  spline S31 degree 5 poles (-10.7975, -4.2396) (-10.7928, -4.2402) (-10.7836, -4.2414) (-10.7697, -4.2432) (-10.7512, -4.2456) (-10.728, -4.2484) (-10.7049, -4.2511) (-10.6819, -4.2537) (-10.6588, -4.2562) (-10.6358, -4.2586) (-10.6127, -4.2609) (-10.5897, -4.2631) (-10.5668, -4.2652) (-10.5438, -4.2672) (-10.5209, -4.269) (-10.498, -4.2708) (-10.4751, -4.2725) (-10.4523, -4.274) (-10.4294, -4.2755) (-10.4066, -4.2768) (-10.3839, -4.2781) (-10.3611, -4.2792) (-10.3384, -4.2802) (-10.3157, -4.2811) (-10.2931, -4.2819) (-10.2704, -4.2826) (-10.2478, -4.2831) (-10.2253, -4.2836) (-10.2027, -4.2839) (-10.1802, -4.2842) (-10.1577, -4.2843) (-10.1353, -4.2843) (-10.1129, -4.2841) (-10.0905, -4.2839) (-10.0682, -4.2835) (-10.0459, -4.283) (-10.0236, -4.2824) (-10.0014, -4.2817) (-9.9792, -4.2808) (-9.9571, -4.2798) (-9.9349, -4.2787) (-9.9129, -4.2775) (-9.8908, -4.2761) (-9.8689, -4.2746) (-9.8469, -4.2729) (-9.825, -4.2712) (-9.8032, -4.2693) (-9.7814, -4.2672) (-9.7596, -4.265) (-9.7379, -4.2627) (-9.7162, -4.2602) (-9.6946, -4.2576) (-9.6731, -4.2548) (-9.6516, -4.2519) (-9.6301, -4.2487) (-9.6088, -4.2455) (-9.5874, -4.2421) (-9.5662, -4.2385) (-9.5449, -4.2348) (-9.5238, -4.2309) (-9.5027, -4.2268) (-9.4817, -4.2225) (-9.4609, -4.2179) (-9.4401, -4.2131) (-9.4194, -4.208) (-9.3988, -4.2028) (-9.3782, -4.1974) (-9.3577, -4.1919) (-9.3372, -4.1863) (-9.317, -4.1803) (-9.2969, -4.1737) (-9.281, -4.1679) (-9.2693, -4.1632) (-9.2616, -4.1598) (-9.2577, -4.1581) knots -1 -1 -1 -1 -1 -1 -0.98571429 -0.97142857 -0.95714286 -0.94285714 -0.92857143 -0.91428571 -0.9 -0.88571429 -0.87142857 -0.85714286 -0.84285714 -0.82857143 -0.81428571 -0.8 -0.78571429 -0.77142857 -0.75714286 -0.74285714 -0.72857143 -0.71428571 -0.7 -0.68571429 -0.67142857 -0.65714286 -0.64285714 -0.62857143 -0.61428571 -0.6 -0.58571429 -0.57142857 -0.55714286 -0.54285714 -0.52857143 -0.51428571 -0.5 -0.48571429 -0.47142857 -0.45714286 -0.44285714 -0.42857143 -0.41428571 -0.4 -0.38571429 -0.37142857 -0.35714286 -0.34285714 -0.32857143 -0.31428571 -0.3 -0.28571429 -0.27142857 -0.25714286 -0.24285714 -0.22857143 -0.21428571 -0.2 -0.18571429 -0.17142857 -0.15714286 -0.14285714 -0.12857143 -0.11428571 -0.1 -0.08571429 -0.07142857 -0.05714286 -0.04285714 -0.02857143 -0.01428571 0 0 0 0 0 0
  line L31 (-9.2577, -4.1581) -> (-9.0202, -4.052)
  arc A63 (-8.8886, -4.1014) -> (-9.0202, -4.052) centre (-8.9794, -4.1433) ccw
  arc A64 (-8.8886, -4.1014) -> (-8.5977, -4.6806) centre (0, 0) ccw
  arc A65 (-8.6367, -4.8156) -> (-8.5977, -4.6806) centre (-8.6855, -4.7284) ccw
  line L32 (-8.6367, -4.8156) -> (-8.8637, -4.9428)
  spline S32 degree 5 poles (-8.8637, -4.9428) (-8.8673, -4.9448) (-8.8747, -4.9491) (-8.8855, -4.9556) (-8.8996, -4.9649) (-8.9168, -4.9771) (-8.9337, -4.9897) (-8.9505, -5.0028) (-8.9671, -5.0159) (-8.9837, -5.0292) (-9.0002, -5.0427) (-9.0166, -5.0562) (-9.0329, -5.07) (-9.0491, -5.084) (-9.0651, -5.0983) (-9.0809, -5.1127) (-9.0967, -5.1274) (-9.1123, -5.1422) (-9.1279, -5.1571) (-9.1434, -5.1722) (-9.1587, -5.1874) (-9.174, -5.2027) (-9.1892, -5.2182) (-9.2044, -5.2338) (-9.2194, -5.2496) (-9.2343, -5.2655) (-9.2491, -5.2815) (-9.2639, -5.2976) (-9.2785, -5.3139) (-9.2931, -5.3303) (-9.3076, -5.3468) (-9.322, -5.3634) (-9.3364, -5.3802) (-9.3506, -5.397) (-9.3648, -5.414) (-9.3789, -5.431) (-9.3929, -5.4482) (-9.4068, -5.4655) (-9.4207, -5.4829) (-9.4345, -5.5004) (-9.4482, -5.518) (-9.4618, -5.5357) (-9.4754, -5.5535) (-9.4889, -5.5714) (-9.5023, -5.5894) (-9.5156, -5.6075) (-9.5289, -5.6257) (-9.5421, -5.6439) (-9.5552, -5.6623) (-9.5682, -5.6808) (-9.5812, -5.6993) (-9.5941, -5.718) (-9.6069, -5.7367) (-9.6197, -5.7555) (-9.6324, -5.7745) (-9.645, -5.7935) (-9.6575, -5.8125) (-9.67, -5.8317) (-9.6824, -5.851) (-9.6947, -5.8703) (-9.7069, -5.8898) (-9.7191, -5.9093) (-9.7312, -5.9289) (-9.7433, -5.9485) (-9.7553, -5.9683) (-9.7672, -5.9881) (-9.779, -6.008) (-9.7907, -6.028) (-9.8024, -6.0481) (-9.8141, -6.0683) (-9.8256, -6.0885) (-9.8348, -6.1047) (-9.8417, -6.1169) (-9.8462, -6.1251) (-9.8485, -6.1292) knots 0 0 0 0 0 0 0.01428571 0.02857143 0.04285714 0.05714286 0.07142857 0.08571429 0.1 0.11428571 0.12857143 0.14285714 0.15714286 0.17142857 0.18571429 0.2 0.21428571 0.22857143 0.24285714 0.25714286 0.27142857 0.28571429 0.3 0.31428571 0.32857143 0.34285714 0.35714286 0.37142857 0.38571429 0.4 0.41428571 0.42857143 0.44285714 0.45714286 0.47142857 0.48571429 0.5 0.51428571 0.52857143 0.54285714 0.55714286 0.57142857 0.58571429 0.6 0.61428571 0.62857143 0.64285714 0.65714286 0.67142857 0.68571429 0.7 0.71428571 0.72857143 0.74285714 0.75714286 0.77142857 0.78571429 0.8 0.81428571 0.82857143 0.84285714 0.85714286 0.87142857 0.88571429 0.9 0.91428571 0.92857143 0.94285714 0.95714286 0.97142857 0.98571429 1 1 1 1 1 1
  arc A66 (-9.8485, -6.1292) -> (-9.5287, -6.6154) centre (0, 0) ccw
  spline S33 degree 5 poles (-9.5287, -6.6154) (-9.5241, -6.6149) (-9.5148, -6.614) (-9.5008, -6.6125) (-9.4823, -6.6105) (-9.4591, -6.6079) (-9.436, -6.6052) (-9.413, -6.6024) (-9.3899, -6.5996) (-9.367, -6.5966) (-9.344, -6.5935) (-9.3212, -6.5903) (-9.2983, -6.5871) (-9.2755, -6.5837) (-9.2528, -6.5803) (-9.2301, -6.5767) (-9.2075, -6.573) (-9.1849, -6.5693) (-9.1623, -6.5654) (-9.1398, -6.5615) (-9.1174, -6.5574) (-9.095, -6.5533) (-9.0727, -6.549) (-9.0504, -6.5447) (-9.0281, -6.5402) (-9.006, -6.5357) (-8.9838, -6.531) (-8.9618, -6.5262) (-8.9398, -6.5214) (-8.9178, -6.5164) (-8.8959, -6.5113) (-8.8741, -6.5061) (-8.8523, -6.5008) (-8.8306, -6.4954) (-8.809, -6.4899) (-8.7874, -6.4843) (-8.7658, -6.4786) (-8.7444, -6.4727) (-8.723, -6.4668) (-8.7017, -6.4607) (-8.6804, -6.4545) (-8.6592, -6.4482) (-8.6381, -6.4418) (-8.6171, -6.4353) (-8.5961, -6.4286) (-8.5752, -6.4218) (-8.5544, -6.4149) (-8.5336, -6.4079) (-8.5129, -6.4008) (-8.4923, -6.3935) (-8.4718, -6.3861) (-8.4514, -6.3786) (-8.4311, -6.3709) (-8.4109, -6.3631) (-8.3907, -6.3551) (-8.3707, -6.347) (-8.3507, -6.3387) (-8.3308, -6.3304) (-8.311, -6.3219) (-8.2914, -6.3132) (-8.2718, -6.3044) (-8.2524, -6.2953) (-8.2331, -6.286) (-8.214, -6.2765) (-8.1951, -6.2668) (-8.1762, -6.257) (-8.1574, -6.247) (-8.1387, -6.237) (-8.1201, -6.2268) (-8.1018, -6.2162) (-8.0837, -6.2052) (-8.0697, -6.196) (-8.0594, -6.1886) (-8.0526, -6.1836) (-8.0493, -6.181) knots -1 -1 -1 -1 -1 -1 -0.98571429 -0.97142857 -0.95714286 -0.94285714 -0.92857143 -0.91428571 -0.9 -0.88571429 -0.87142857 -0.85714286 -0.84285714 -0.82857143 -0.81428571 -0.8 -0.78571429 -0.77142857 -0.75714286 -0.74285714 -0.72857143 -0.71428571 -0.7 -0.68571429 -0.67142857 -0.65714286 -0.64285714 -0.62857143 -0.61428571 -0.6 -0.58571429 -0.57142857 -0.55714286 -0.54285714 -0.52857143 -0.51428571 -0.5 -0.48571429 -0.47142857 -0.45714286 -0.44285714 -0.42857143 -0.41428571 -0.4 -0.38571429 -0.37142857 -0.35714286 -0.34285714 -0.32857143 -0.31428571 -0.3 -0.28571429 -0.27142857 -0.25714286 -0.24285714 -0.22857143 -0.21428571 -0.2 -0.18571429 -0.17142857 -0.15714286 -0.14285714 -0.12857143 -0.11428571 -0.1 -0.08571429 -0.07142857 -0.05714286 -0.04285714 -0.02857143 -0.01428571 0 0 0 0 0 0
  line L33 (-8.0493, -6.181) -> (-7.8426, -6.023)
  arc A67 (-7.7031, -6.0407) -> (-7.8426, -6.023) centre (-7.7818, -6.1024) ccw
  arc A68 (-7.7031, -6.0407) -> (-7.2866, -6.5372) centre (0, 0) ccw
  arc A69 (-7.2933, -6.6776) -> (-7.2866, -6.5372) centre (-7.361, -6.6039) ccw
  line L34 (-7.2933, -6.6776) -> (-7.4849, -6.8537)
  spline S34 degree 5 poles (-7.4849, -6.8537) (-7.488, -6.8565) (-7.4941, -6.8623) (-7.5031, -6.8712) (-7.5147, -6.8834) (-7.5287, -6.8993) (-7.5422, -6.9155) (-7.5555, -6.932) (-7.5687, -6.9487) (-7.5817, -6.9655) (-7.5947, -6.9823) (-7.6075, -6.9993) (-7.6202, -7.0165) (-7.6327, -7.0338) (-7.645, -7.0514) (-7.6571, -7.0691) (-7.669, -7.087) (-7.6808, -7.105) (-7.6925, -7.1231) (-7.7041, -7.1414) (-7.7156, -7.1597) (-7.7269, -7.1782) (-7.7381, -7.1967) (-7.7492, -7.2154) (-7.7602, -7.2342) (-7.7711, -7.2531) (-7.7818, -7.2721) (-7.7924, -7.2912) (-7.8029, -7.3105) (-7.8133, -7.3298) (-7.8237, -7.3492) (-7.8339, -7.3687) (-7.8439, -7.3883) (-7.8539, -7.4079) (-7.8638, -7.4277) (-7.8736, -7.4476) (-7.8833, -7.4675) (-7.8928, -7.4876) (-7.9023, -7.5077) (-7.9117, -7.5279) (-7.921, -7.5482) (-7.9302, -7.5685) (-7.9393, -7.589) (-7.9483, -7.6095) (-7.9572, -7.6301) (-7.966, -7.6508) (-7.9747, -7.6715) (-7.9833, -7.6924) (-7.9918, -7.7133) (-8.0002, -7.7342) (-8.0086, -7.7553) (-8.0168, -7.7764) (-8.025, -7.7976) (-8.0331, -7.8189) (-8.041, -7.8402) (-8.0489, -7.8616) (-8.0567, -7.883) (-8.0644, -7.9046) (-8.072, -7.9262) (-8.0796, -7.9478) (-8.087, -7.9696) (-8.0944, -7.9914) (-8.1016, -8.0132) (-8.1088, -8.0351) (-8.1159, -8.0571) (-8.1229, -8.0792) (-8.1298, -8.1013) (-8.1367, -8.1234) (-8.1434, -8.1457) (-8.1501, -8.168) (-8.1567, -8.1903) (-8.1619, -8.2082) (-8.1657, -8.2217) (-8.1683, -8.2307) (-8.1696, -8.2352) knots 0 0 0 0 0 0 0.01428571 0.02857143 0.04285714 0.05714286 0.07142857 0.08571429 0.1 0.11428571 0.12857143 0.14285714 0.15714286 0.17142857 0.18571429 0.2 0.21428571 0.22857143 0.24285714 0.25714286 0.27142857 0.28571429 0.3 0.31428571 0.32857143 0.34285714 0.35714286 0.37142857 0.38571429 0.4 0.41428571 0.42857143 0.44285714 0.45714286 0.47142857 0.48571429 0.5 0.51428571 0.52857143 0.54285714 0.55714286 0.57142857 0.58571429 0.6 0.61428571 0.62857143 0.64285714 0.65714286 0.67142857 0.68571429 0.7 0.71428571 0.72857143 0.74285714 0.75714286 0.77142857 0.78571429 0.8 0.81428571 0.82857143 0.84285714 0.85714286 0.87142857 0.88571429 0.9 0.91428571 0.92857143 0.94285714 0.95714286 0.97142857 0.98571429 1 1 1 1 1 1
  arc A70 (-8.1696, -8.2352) -> (-7.7462, -8.6346) centre (0, 0) ccw
  spline S35 degree 5 poles (-7.7462, -8.6346) (-7.7418, -8.633) (-7.733, -8.63) (-7.7198, -8.6253) (-7.7022, -8.6191) (-7.6803, -8.6112) (-7.6584, -8.6033) (-7.6366, -8.5952) (-7.6149, -8.5871) (-7.5932, -8.5789) (-7.5716, -8.5707) (-7.5501, -8.5623) (-7.5286, -8.5539) (-7.5072, -8.5453) (-7.4859, -8.5367) (-7.4646, -8.528) (-7.4434, -8.5193) (-7.4223, -8.5104) (-7.4012, -8.5014) (-7.3803, -8.4924) (-7.3594, -8.4833) (-7.3385, -8.4741) (-7.3178, -8.4648) (-7.2971, -8.4554) (-7.2765, -8.446) (-7.256, -8.4364) (-7.2355, -8.4268) (-7.2152, -8.4171) (-7.1949, -8.4072) (-7.1746, -8.3973) (-7.1545, -8.3873) (-7.1345, -8.3773) (-7.1145, -8.3671) (-7.0946, -8.3568) (-7.0748, -8.3465) (-7.0551, -8.336) (-7.0355, -8.3255) (-7.016, -8.3149) (-6.9965, -8.3041) (-6.9772, -8.2933) (-6.9579, -8.2824) (-6.9387, -8.2714) (-6.9197, -8.2603) (-6.9007, -8.249) (-6.8818, -8.2377) (-6.8631, -8.2263) (-6.8444, -8.2148) (-6.8258, -8.2032) (-6.8073, -8.1915) (-6.789, -8.1797) (-6.7707, -8.1677) (-6.7526, -8.1557) (-6.7346, -8.1435) (-6.7167, -8.1312) (-6.699, -8.1188) (-6.6813, -8.1063) (-6.6638, -8.0937) (-6.6464, -8.081) (-6.6291, -8.0681) (-6.6119, -8.0552) (-6.5949, -8.0421) (-6.5781, -8.0288) (-6.5615, -8.0153) (-6.5451, -8.0016) (-6.5289, -7.9878) (-6.5128, -7.9739) (-6.4969, -7.9599) (-6.481, -7.9458) (-6.4653, -7.9315) (-6.4498, -7.9171) (-6.4348, -7.9022) (-6.4233, -7.8899) (-6.4149, -7.8804) (-6.4095, -7.874) (-6.4069, -7.8707) knots -1 -1 -1 -1 -1 -1 -0.98571429 -0.97142857 -0.95714286 -0.94285714 -0.92857143 -0.91428571 -0.9 -0.88571429 -0.87142857 -0.85714286 -0.84285714 -0.82857143 -0.81428571 -0.8 -0.78571429 -0.77142857 -0.75714286 -0.74285714 -0.72857143 -0.71428571 -0.7 -0.68571429 -0.67142857 -0.65714286 -0.64285714 -0.62857143 -0.61428571 -0.6 -0.58571429 -0.57142857 -0.55714286 -0.54285714 -0.52857143 -0.51428571 -0.5 -0.48571429 -0.47142857 -0.45714286 -0.44285714 -0.42857143 -0.41428571 -0.4 -0.38571429 -0.37142857 -0.35714286 -0.34285714 -0.32857143 -0.31428571 -0.3 -0.28571429 -0.27142857 -0.25714286 -0.24285714 -0.22857143 -0.21428571 -0.2 -0.18571429 -0.17142857 -0.15714286 -0.14285714 -0.12857143 -0.11428571 -0.1 -0.08571429 -0.07142857 -0.05714286 -0.04285714 -0.02857143 -0.01428571 0 0 0 0 0 0
  line L35 (-6.4069, -7.8707) -> (-6.2422, -7.6692)
  arc A71 (-6.1024, -7.6543) -> (-6.2422, -7.6692) centre (-6.1648, -7.7325) ccw
  arc A72 (-6.1024, -7.6543) -> (-5.5826, -8.0414) centre (0, 0) ccw
  arc A73 (-5.5568, -8.1795) -> (-5.5826, -8.0414) centre (-5.6396, -8.1235) ccw
  line L36 (-5.5568, -8.1795) -> (-5.7025, -8.395)
  spline S36 degree 5 poles (-5.7025, -8.395) (-5.7049, -8.3985) (-5.7095, -8.4056) (-5.7163, -8.4163) (-5.7247, -8.4309) (-5.7346, -8.4495) (-5.7441, -8.4685) (-5.7532, -8.4876) (-5.7622, -8.5068) (-5.771, -8.5262) (-5.7797, -8.5456) (-5.7883, -8.5651) (-5.7967, -8.5847) (-5.8048, -8.6045) (-5.8128, -8.6244) (-5.8204, -8.6444) (-5.8279, -8.6646) (-5.8353, -8.6848) (-5.8425, -8.7052) (-5.8495, -8.7256) (-5.8565, -8.7461) (-5.8632, -8.7666) (-5.8699, -8.7873) (-5.8764, -8.808) (-5.8827, -8.8288) (-5.8889, -8.8497) (-5.895, -8.8707) (-5.9009, -8.8918) (-5.9067, -8.9129) (-5.9124, -8.9341) (-5.9179, -8.9553) (-5.9234, -8.9767) (-5.9287, -8.998) (-5.9338, -9.0195) (-5.9389, -9.041) (-5.9438, -9.0626) (-5.9486, -9.0842) (-5.9533, -9.1059) (-5.9579, -9.1277) (-5.9624, -9.1495) (-5.9668, -9.1714) (-5.971, -9.1933) (-5.9751, -9.2153) (-5.9791, -9.2374) (-5.9831, -9.2595) (-5.9868, -9.2816) (-5.9905, -9.3038) (-5.9941, -9.3261) (-5.9976, -9.3484) (-6.001, -9.3707) (-6.0042, -9.3931) (-6.0074, -9.4156) (-6.0104, -9.4381) (-6.0134, -9.4606) (-6.0162, -9.4832) (-6.019, -9.5059) (-6.0216, -9.5286) (-6.0241, -9.5513) (-6.0266, -9.5741) (-6.0289, -9.5969) (-6.0311, -9.6197) (-6.0333, -9.6426) (-6.0353, -9.6656) (-6.0372, -9.6886) (-6.039, -9.7116) (-6.0408, -9.7347) (-6.0424, -9.7578) (-6.044, -9.7809) (-6.0454, -9.8041) (-6.0467, -9.8273) (-6.048, -9.8506) (-6.0489, -9.8692) (-6.0496, -9.8832) (-6.05, -9.8926) (-6.0502, -9.8972) knots 0 0 0 0 0 0 0.01428571 0.02857143 0.04285714 0.05714286 0.07142857 0.08571429 0.1 0.11428571 0.12857143 0.14285714 0.15714286 0.17142857 0.18571429 0.2 0.21428571 0.22857143 0.24285714 0.25714286 0.27142857 0.28571429 0.3 0.31428571 0.32857143 0.34285714 0.35714286 0.37142857 0.38571429 0.4 0.41428571 0.42857143 0.44285714 0.45714286 0.47142857 0.48571429 0.5 0.51428571 0.52857143 0.54285714 0.55714286 0.57142857 0.58571429 0.6 0.61428571 0.62857143 0.64285714 0.65714286 0.67142857 0.68571429 0.7 0.71428571 0.72857143 0.74285714 0.75714286 0.77142857 0.78571429 0.8 0.81428571 0.82857143 0.84285714 0.85714286 0.87142857 0.88571429 0.9 0.91428571 0.92857143 0.94285714 0.95714286 0.97142857 0.98571429 1 1 1 1 1 1
  arc A74 (-6.0502, -9.8972) -> (-5.5462, -10.1882) centre (0, 0) ccw
  spline S37 degree 5 poles (-5.5462, -10.1882) (-5.5422, -10.1857) (-5.5344, -10.1807) (-5.5226, -10.1731) (-5.5069, -10.163) (-5.4874, -10.1503) (-5.4679, -10.1375) (-5.4486, -10.1247) (-5.4293, -10.1118) (-5.4101, -10.0988) (-5.391, -10.0858) (-5.3719, -10.0727) (-5.353, -10.0595) (-5.3342, -10.0463) (-5.3154, -10.033) (-5.2967, -10.0196) (-5.2781, -10.0062) (-5.2596, -9.9927) (-5.2412, -9.9791) (-5.2229, -9.9655) (-5.2046, -9.9518) (-5.1865, -9.9381) (-5.1684, -9.9242) (-5.1505, -9.9103) (-5.1326, -9.8964) (-5.1148, -9.8824) (-5.0971, -9.8683) (-5.0796, -9.8541) (-5.0621, -9.8399) (-5.0447, -9.8256) (-5.0274, -9.8112) (-5.0102, -9.7968) (-4.9931, -9.7823) (-4.9762, -9.7677) (-4.9593, -9.7531) (-4.9425, -9.7384) (-4.9259, -9.7236) (-4.9093, -9.7087) (-4.8929, -9.6938) (-4.8765, -9.6788) (-4.8603, -9.6637) (-4.8442, -9.6486) (-4.8282, -9.6334) (-4.8123, -9.6181) (-4.7966, -9.6027) (-4.7809, -9.5873) (-4.7654, -9.5718) (-4.75, -9.5562) (-4.7348, -9.5406) (-4.7196, -9.5248) (-4.7046, -9.509) (-4.6898, -9.4931) (-4.6751, -9.4771) (-4.6605, -9.461) (-4.6461, -9.4449) (-4.6318, -9.4286) (-4.6176, -9.4123) (-4.6036, -9.3959) (-4.5898, -9.3794) (-4.5761, -9.3629) (-4.5626, -9.3462) (-4.5493, -9.3294) (-4.5362, -9.3124) (-4.5234, -9.2954) (-4.5108, -9.2782) (-4.4984, -9.2609) (-4.4861, -9.2436) (-4.4739, -9.2262) (-4.4619, -9.2087) (-4.4502, -9.1911) (-4.439, -9.1732) (-4.4306, -9.1586) (-4.4247, -9.1474) (-4.4209, -9.1399) (-4.419, -9.1361) knots -1 -1 -1 -1 -1 -1 -0.98571429 -0.97142857 -0.95714286 -0.94285714 -0.92857143 -0.91428571 -0.9 -0.88571429 -0.87142857 -0.85714286 -0.84285714 -0.82857143 -0.81428571 -0.8 -0.78571429 -0.77142857 -0.75714286 -0.74285714 -0.72857143 -0.71428571 -0.7 -0.68571429 -0.67142857 -0.65714286 -0.64285714 -0.62857143 -0.61428571 -0.6 -0.58571429 -0.57142857 -0.55714286 -0.54285714 -0.52857143 -0.51428571 -0.5 -0.48571429 -0.47142857 -0.45714286 -0.44285714 -0.42857143 -0.41428571 -0.4 -0.38571429 -0.37142857 -0.35714286 -0.34285714 -0.32857143 -0.31428571 -0.3 -0.28571429 -0.27142857 -0.25714286 -0.24285714 -0.22857143 -0.21428571 -0.2 -0.18571429 -0.17142857 -0.15714286 -0.14285714 -0.12857143 -0.11428571 -0.1 -0.08571429 -0.07142857 -0.05714286 -0.04285714 -0.02857143 -0.01428571 0 0 0 0 0 0
  line L37 (-4.419, -9.1361) -> (-4.3053, -8.9021)
  arc A75 (-4.1727, -8.8553) -> (-4.3053, -8.9021) centre (-4.2154, -8.9458) ccw
  arc A76 (-4.1727, -8.8553) -> (-3.5776, -9.112) centre (0, 0) ccw
  arc A77 (-3.5207, -9.2405) -> (-3.5776, -9.112) centre (-3.6142, -9.2051) ccw
  line L38 (-3.5207, -9.2405) -> (-3.6128, -9.4838)